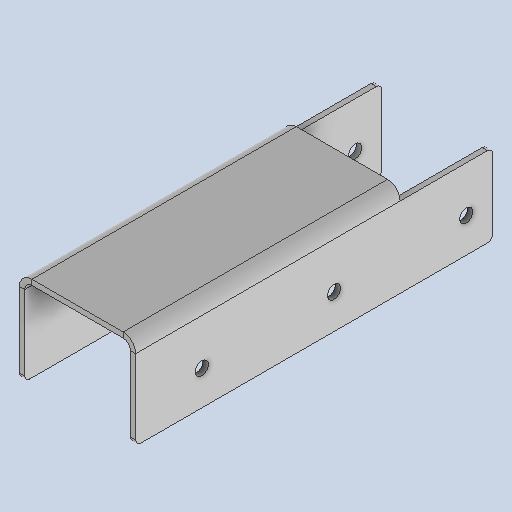
# Autodesk Inventor part: NDM 4.0.8 bracket1
Saved by Autodesk Inventor 2025 (Build 290162010, 162A)
## iProperties
Created: 2024-06-12
Part Number: NDM 4.0.8 bracket1
Material: Stainless Steel
Document SubType Name: Sheet Metal
Designer: admin
Density: 8 g/cm^3
Sheet Metal Rule: AISI304 2mm Die16
Appearance: Default
Flat Pattern Width: 10.6404 cm
Flat Pattern Length: 13.5 cm
Flat Pattern Area: 143.645 cm^2
Sheet Metal Width: 106,404 mm
Sheet Metal Length: 135,000 mm
Sheet Metal Area: 14364,537 mm^2
Description: 2mm
Mass: 202.762 g
Surface Area: 266.306 cm^2
Volume: 25.3453 cm^3
Author: admin
Revision Number: 8
Autodesk Inventor part; units mm, degrees
note: some values were not read from the file. Chosen so that the rebuilt part matches the saved one: flange form of "Plate2".
ref_plane "YZ Plane" through (0, 0, 0) normal (1, 0, 0) x (0, 1, 0)
ref_plane "XZ Plane" through (0, 0, 0) normal (0, 1, 0) x (-1, 0, 0)
ref_plane "XY Plane" through (0, 0, 0) normal (0, 0, 1) x (1, 0, 0)
sketch "Sketch1" plane through (0, 0, 0) normal (0, 0, 1) x (1, 0, 0)
  line L0 (-20, 0) -> (20, 0)
  line L1 (20, 0) -> (20, -100)
  line L2 (20, -100) -> (-20, -100)
  line L3 (-20, -100) -> (-20, 0)
  point P0 (0, 0)
  point P1 (0, 0)
  dimension "d0" = 40
  dimension "d1" = 100
  measures "d0" distance of L1.end L2.end
  measures "d1" distance of L0.end L1.end
extrude "Plate1" add sketch "Sketch1" along normal blind 2
sketch "Sketch2" plane through (20, -100, 0) normal (1, 0, 0) x (0, 1, 0)
  line L0 (100, 0) -> (0, 0)
  line L1 (0, 0) -> (0, -33)
  line L2 (0, -33) -> (100, -33)
  line L3 (100, -33) -> (100, 0)
  constraints: 6 end point, 1 horizontal, 1 perpendicular, 1 vertical
edge flange "Flange1" height 35 angle 90 thickness 2 bend radius 2.75 thickness toward (1, 0, 0) relief round relief width 2 relief depth 1 corner gap 2.75 corner form 0 edges at (20, -50, 0) (-20, -50, 0) wall of the first edge with corners at (20, 0, 0) (20, -100, 0) (20, -100, -33) (20, 0, -33)
bend "Bend1"
corner "Corner1"
sketch "Sketch5" plane through (-17.25, 0, 0) normal (0, 1, 0) x (1, 0, 0)
  line L0 (-4.75, 2.75) -> (-2.75, 2.75) projected
  line L1 (-2.75, 2.75) -> (-2.75, 33) projected
  line L2 (-2.75, 33) -> (-4.75, 33) projected
  line L3 (-4.75, 33) -> (-4.75, 2.75) projected
  line L4 (37.25, 2.75) -> (39.25, 2.75) projected
  line L5 (39.25, 2.75) -> (39.25, 33) projected
  line L6 (37.25, 33) -> (39.25, 33) projected
  line L7 (37.25, 2.75) -> (37.25, 33) projected
  point P0 (17.25, 0)
extrude "Extrusion2" add sketch "Sketch5" along normal blind 35
sketch "Sketch3" plane through (0, 0, 0) normal (1, 0, 0) x (0, 1, 0)
  line L0 (0, -33) -> (-100, -33) projected
  line L1 (-75, -20) -> (-75, -20) construction
  line L2 (-77.5, -20) -> (-77.5, -20)
  line L3 (-72.5, -20) -> (-72.5, -20)
  arc A0 (-72.5, -20) -> (-77.5, -20) centre (-75, -20) ccw
  arc A1 (-77.5, -20) -> (-72.5, -20) centre (-75, -20) ccw
  line L4 (-100, -2.75) -> (-100, -33) projected
  point P0 (0, 0)
  dimension "d14" = 0
  dimension "d15" = 13
  dimension "d17" = 2.5
  dimension "d18" = 25
  constraints: 8 end point, 4 point on circle, 4 tangent, 2 centre point, 1 midpoint, 1 parallel, 1 vertical
  measures "d14" distance of L1.start L1.end
  measures "d15" distance from line of L0 L1.start
  measures "d17" radius of A1
  measures "d18" distance from line of L4 point (-75, -20)
extrude "Extrusion1" cut sketch "Sketch3" along normal through all both and the other way through all
pattern_linear "Rectangular Pattern1" count 3 spacing 50 along (0, 1, 0) of "Extrusion1"
fillet "Fillet1" radius 2 6 edges at (21, 35, -2.75) (-21, 35, -2.75) (-21, 35, -33) (21, 35, -33) (21, -100, -33) (-21, -100, -33)
equation "\"d2\" = Thickness"
equation "\"d3\" = BendReliefWidth"
equation "\"d4\" = BendReliefDepth"
equation "\"d5\" = MinimumRemnant"
equation "\"d6\" = TransitionRadius"
equation "\"d9\" = BendRadius"
equation "\"d10\" = CornerReliefSize"
equation "\"d11\" = GapSize"
equation "\"d12\" = JacobiRadiusSize"
equation "\"BendReliefWidth\" = Thickness"
equation "\"BendReliefDepth\" = 0.5 * Thickness"
equation "\"CornerReliefSize\" = 4 * Thickness"
equation "\"MinimumRemnant\" = 2 * Thickness"
equation "\"TransitionRadius\" = BendRadius"
equation "\"JacobiRadiusSize\" = BendRadius"
equation "\"GapSize\" = Thickness"
equation "\"Thickness\" = 2"
equation "\"BendRadius\" = 2.75"
body "Solid1"
